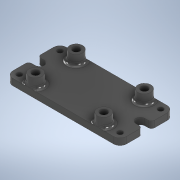
# Autodesk Inventor part: rpiCamMount
Saved by Autodesk Inventor 2020 (Build 240168000, 168)
## iProperties
Created: 2019-08-05
Part Number: rpiCamMount
Material: Generic
Document SubType Name: Modeling
Designer: n10208577
Density: 1 g/cm^3
Appearance: Default
Author: n10208577
Autodesk Inventor part; units mm, degrees
ref_plane "YZ Plane" through (0, 0, 0) normal (1, 0, 0) x (0, 1, 0)
ref_plane "XZ Plane" through (0, 0, 0) normal (0, 1, 0) x (-1, 0, 0)
ref_plane "XY Plane" through (0, 0, 0) normal (0, 0, 1) x (1, 0, 0)
sketch "Sketch1" plane through (0, 0, 0) normal (0, 1, 0) x (-1, 0, 0)
  line L0 (0, 0) -> (-35, 0)
  line L1 (-35, -16.5) -> (0, -16.5)
  line L2 (0, 0) -> (0, -2)
  line L3 (0, -2) -> (-2, -2)
  circle A0 centre (-2, -2) radius 0.8
  line L4 (-2, -2) -> (-33, -2)
  line L5 (-33, -14.5) -> (-2, -14.5)
  circle A1 centre (-2, -14.5) radius 0.8
  circle A2 centre (-33, -14.5) radius 0.8
  circle A3 centre (-33, -2) radius 0.8
  arc A4 (-2, -6.85) -> (-2, -9.65) centre (-2, -8.25) ccw
  arc A5 (-33, -9.65) -> (-33, -6.85) centre (-33, -8.25) ccw
  line L6 (-2, -6.85) -> (0, -6.85)
  line L7 (-2, -9.65) -> (0, -9.65)
  line L8 (-33, -9.65) -> (-35, -9.65)
  line L9 (-33, -6.85) -> (-35, -6.85)
  line L10 (-33, -2) -> (-33, -6.85)
  line L11 (-33, -9.65) -> (-33, -14.5)
  line L12 (-2, -14.5) -> (-2, -9.65)
  line L13 (-2, -6.85) -> (-2, -2)
  line L14 (0, -16.5) -> (0, -9.65)
  line L15 (0, -6.85) -> (0, 0)
  line L16 (-35, 0) -> (-35, -6.85)
  line L17 (-35, -9.65) -> (-35, -16.5)
  dimension "d0" = 35
  dimension "d1" = 16.5
  dimension "d2" = 2
  dimension "d3" = 2
  dimension "d4" = 1.6
  dimension "d5" = 31
  dimension "d6" = 12.5
  dimension "d7" = 1.6
  dimension "d8" = 1.6
  dimension "d9" = 1.6
  dimension "d10" = 2.8
  dimension "d11" = 2.8
  constraints: 36 end point, 10 parallel, 9 perpendicular, 6 centre point, 4 coincident, 4 point on circle, 3 point on line, 2 horizontal, 2 tangent
  measures "d0" distance of L1.end L1.start
  measures "d1" distance of L1.start L0.end
  measures "d2" distance of L0.start L2.end
  measures "d3" distance of L2.end L3.end
  measures "d4" diameter of A0
  measures "d5" distance of L5.end L5.start
  measures "d6" distance of L5.start L4.end
  measures "d7" diameter of A1
  measures "d8" diameter of A2
  measures "d9" diameter of A3
  measures "d10" diameter of A4
  measures "d11" diameter of A5
extrude "Extrusion1" add sketch "Sketch1" along normal blind 2 contours L2 L3 A0 L4 A3 L10 L9 L16 L0 | L15 L6 L13 A0 L3 | L10 A3 L4 A0 L13 A4 L12 A1 L5 A2 L11 A5 | L11 A2 L5 A1 L12 L7 L14 L1 L17 L8
sketch "Sketch2" plane through (0, 2, 0) normal (0, 1, 0) x (1, 0, 0)
  line L0 (35, 16.5) -> (0, 16.5) projected
  line L1 (0, 16.5) -> (0, 9.65) projected
  line L2 (0, 9.65) -> (2, 9.65) projected
  arc A0 (2, 6.85) -> (2, 9.65) centre (2, 8.25) ccw projected
  line L3 (2, 6.85) -> (0, 6.85) projected
  line L4 (0, 6.85) -> (0, 0) projected
  line L5 (0, 0) -> (35, 0) projected
  line L6 (35, 0) -> (35, 6.85) projected
  line L7 (35, 6.85) -> (33, 6.85) projected
  arc A1 (33, 9.65) -> (33, 6.85) centre (33, 8.25) ccw projected
  line L8 (33, 9.65) -> (35, 9.65) projected
  line L9 (35, 9.65) -> (35, 16.5) projected
  circle A2 centre (2, 2) radius 0.8 projected
  circle A3 centre (33, 2) radius 0.8 projected
  circle A4 centre (33, 14.5) radius 0.8 projected
  circle A5 centre (2, 14.5) radius 0.8 projected
  line L10 (0, 0) -> (35, 0) projected
  line L11 (17.5, 0) -> (17.5, 2)
  line L12 (17.5, 2) -> (17.5, 14.5)
  line L13 (17.5, 2) -> (7, 2)
  line L14 (17.5, 2) -> (28, 2)
  line L15 (17.5, 14.5) -> (28, 14.5)
  line L16 (17.5, 14.5) -> (7, 14.5)
  circle A6 centre (7, 14.5) radius 1.1
  circle A7 centre (7, 2) radius 1.1
  circle A8 centre (28, 2) radius 1.1
  circle A9 centre (28, 14.5) radius 1.1
  circle A10 centre (7, 2) radius 2
  circle A11 centre (7, 14.5) radius 2
  circle A12 centre (28, 14.5) radius 2
  circle A13 centre (28, 2) radius 2
  dimension "d14" = 2
  dimension "d15" = 10.5
  dimension "d16" = 10.5
  dimension "d17" = 10.5
  dimension "d18" = 10.5
  dimension "d19" = 2.2
  dimension "d20" = 2.2
  dimension "d21" = 2.2
  dimension "d22" = 2.2
  dimension "d23" = 4
  dimension "d24" = 4
  dimension "d25" = 4
  dimension "d26" = 4
  constraints: 12 end point, 8 centre point, 8 coincident, 4 horizontal, 1 midpoint, 1 perpendicular, 1 point on line
  measures "d14" distance of L11.start L11.end
  measures "d15" distance of L11.end L13.end
  measures "d16" distance of L11.end L14.end
  measures "d17" distance of L12.end L15.end
  measures "d18" distance of L12.end L16.end
  measures "d19" diameter of A6
  measures "d20" diameter of A7
  measures "d21" diameter of A8
  measures "d22" diameter of A9
  measures "d23" diameter of A10
  measures "d24" diameter of A11
  measures "d25" diameter of A12
  measures "d26" diameter of A13
extrude "Extrusion2" add sketch "Sketch2" along normal blind 3 contours A12 | A11 | A10 | A13
fillet "Fillet1" radius 2 4 edges at (35, 1, 0) (35, 1, -16.5) (0, 1, -16.5) (0, 1, 0)
fillet "Fillet2" radius 1 4 edges at (0, 1, -6.85) (0, 1, -9.65) (35, 1, -6.85) (35, 1, -9.65)
fillet "Fillet3" radius 1 8 edges at (8.4142, 2, -0.5858) (5.5858, 2, -3.4142) (29.4142, 2, -0.5858) (26.5858, 2, -3.4142) (26.5858, 2, -13.0858) (29.4142, 2, -15.9142) (5.5858, 2, -13.0858) (8.4142, 2, -15.9142)
body "Solid1"
